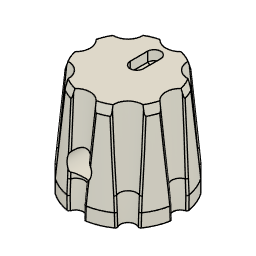
CHORDS Knob 1 (Autodesk Fusion 360 design; units mm, degrees)
Autodesk Fusion 360 part; units mm, degrees
sketch "Sketch1" plane through (0, 0, 0) normal (0, 1, 0) x (1, 0, 0)
  circle A0 centre (0, 0) radius 3
  line L0 (0, 0) -> (0, 3) construction
  line L1 (0, 3) -> (0, -1.6) construction
  line L2 (0, -1.6) -> (-2.5377, -1.6)
  line L3 (0, -1.6) -> (2.5377, -1.6)
  circle A1 centre (0, 0) radius 3.17
  line L4 (0, -1.72) -> (2.5377, -1.72)
  line L5 (0, -1.72) -> (-2.5377, -1.72)
  circle A2 centre (0, 0) radius 4.5
  circle A3 centre (0, 0) radius 6
  line L6 (0, 6) -> (0, 4.5) construction
  circle A4 centre (0, 6) radius 0.875
  circle A5 centre (-4.2426, 4.2426) radius 0.875
  circle A6 centre (-6, 0) radius 0.875
  circle A7 centre (-4.2426, -4.2426) radius 0.875
  circle A8 centre (0, -6) radius 0.875
  circle A9 centre (4.2426, -4.2426) radius 0.875
  circle A10 centre (6, 0) radius 0.875
  line L7 (2.5377, -1.72) -> (2.9, -1.72)
  line L8 (-2.5377, -1.72) -> (-2.8, -1.72)
  circle A11 centre (4.2426, 4.2426) radius 0.875
  line L9 (0, 0) -> (0, 3) construction
  line L10 (-0.75, 3) -> (-0.75, 1)
  arc A12 (-0.75, 1) -> (0.75, 1) centre (0, 1) ccw
  line L11 (0.75, 1) -> (0.75, 3)
  arc A13 (0.75, 3) -> (-0.75, 3) centre (0, 3) ccw
  line L12 (0, 3) -> (0, 1) construction
  dimension "d1" = 6
  dimension "d3" = 4.6
  dimension "d4" = 0.17
  dimension "d5" = 0.12
  dimension "d6" = 9
  dimension "d7" = 1.5
  dimension "d10" = 1.75
  dimension "d12" = 360
  dimension "d62" = 3
  dimension "d63" = 2
  dimension "d64" = 1.5
  constraint coincident A0.centre L0.start
  constraint coincident A0 L0.end
  constraint vertical L0
  constraint parallel L0 L1
  constraint coincident A0 L2.end
  constraint perpendicular L1 L2
  constraint coincident A0 L3.end
  constraint perpendicular L1 L3
  constraint concentric A0 A2
  constraint coincident A3 L6.start
  constraint coincident A2 L6.end
  constraint vertical L6
  constraint coincident L6.start A4.centre
  constraint parallel L4 L7
  constraint parallel L5 L8
  constraint parallel L1 L9
  constraint tangent L10 A12
  constraint tangent A12 L11
  constraint parallel L10 L11
  constraint tangent L11 A13
  constraint tangent L10 A13
  constraint coincident L9 A12.centre
  constraint coincident L0.end L1.start
  measures "d1" diameter of A0
  measures "d3" distance of L0.end L1.end
  measures "d6" diameter of A2
  measures "d10" diameter of A4
  measures "d62" distance of A0.centre L0.end
  measures "d63" distance of L0.end A12.centre
  measures "d64" diameter of A12
extrude "Extrude1" add sketch "Sketch1" along normal blind 10 draft -4.5 contours A0 L2 L3 L10 A12 L11 | A0 A1 L4 L7 L11 A13 | A0 L2 L3 L4 L5 | A0 A1 L4 L5 L7 L8 | A0 L4 L5 | A0 L10 A12 L11 | A0 A1 L10 L11 A13 | A0 A1 L5 L8 L10 A13 | A1 A13 | A2 | A3 A4 A5 A6 A7 A8 A9 A10 A11
sketch "Sketch2" plane through (0, 0, 0) normal (0, 0, 1) x (1, 0, 0)
  line L0 (0, 0) -> (0, 3.2) construction
  circle A0 centre (0, 3.2) radius 1.4
  dimension "d21" = 2.8
  constraint coincident L0.start origin
  constraint vertical L0
  constraint coincident L0.end A0.centre
  measures "d21" diameter of A0
extrude "Extrude5" cut sketch "Sketch1" along normal blind 8 contours A0 L2 L3 L10 A12 L11 | A0 A1 L4 L7 L11 A13 | A0 L2 L3 L4 L5 | A0 L10 A12 L11 | A0 A1 L10 L11 A13 | A0 A1 L5 L8 L10 A13
chamfer "Chamfer2" distance 1 distance2 0.2 8 edges at (4.8162, 10, 1.9949) (1.9949, 10, 4.8162) (-1.9949, 10, 4.8162) (-4.8162, 10, 1.9949) (-4.8162, 10, -1.9949) (-1.9949, 10, -4.8162) (1.9949, 10, -4.8162) (4.8162, 10, -1.9949) measured on face at (5.0774, 6.4078, 2.1031) measured on face at (2.1031, 6.4078, 5.0774) measured on face at (-2.1031, 6.4078, 5.0774) measured on face at (-5.0774, 6.4078, 2.1031) measured on face at (-5.0774, 6.4078, -2.1031) measured on face at (-2.1031, 6.4078, -5.0774) measured on face at (2.1031, 6.4078, -5.0774) measured on face at (5.0774, 6.4078, -2.1031)
extrude "Extrude7" cut sketch "Sketch1" against normal blind 1.5 from surface at 10 contours A0 L10 A12 L11 | A0 A1 L10 L11 A13 | A1 A13
chamfer "Chamfer4" distance 0.4 distance2 0.75 4 edges at (-0.75, 8.5, -2) (0, 8.5, -3.75) (0.75, 8.5, -2) (0, 8.5, -0.25) measured on face at (-0.75, 9.5, -2.3333) measured on face at (0.64, 9, -3.3911) measured on face at (0.75, 9.5, -1.6667) measured on face at (0.5745, 9.5, -0.5179)
extrude "Extrude8" cut sketch "Sketch2" along normal blind 10
extrude "Extrude9" cut sketch "Sketch1" along normal blind 1 contours A0 A1 L4 L5 L7 L8 | A0 L4 L5
chamfer "Chamfer5" distance 0.4 distance2 1 1 edges at (-2.9555, 0, 1.1463) measured on face at (-4.5973, 0, 1.3986)
fillet "Fillet7" radius 1 2 edges at (2.6628, 4.5, 1.72) (-2.6628, 4.5, 1.72)
extrude "Extrude10" add 1 faces at (1.1929, 0, -4.8108) along direction (0, -1, 0) blind 1.5
fillet "Fillet8" radius 40 8 edges at (0, 0, 5.125) (-3.6239, 0, 3.6239) (-5.125, 0, 0) (-3.6239, 0, -3.6239) (0, 0, -5.125) (3.6239, 0, -3.6239) (5.125, 0, 0) (3.6239, 0, 3.6239)
fillet "Fillet3" radius 0.2 50 edges at (3.0348, 5.2493, 4.6908) (3.4859, 0.7834, 4.8076) (1.2253, 6.5121, 5.3489) (0.9973, 1.9012, 5.7647) (0.9346, 0.7833, 5.8643) (-1.2255, 6.515, 5.3487) (-0.9973, 1.9013, 5.7647) (-0.9346, 0.7834, 5.8643) (-3.0357, 5.2413, 4.691) (-3.4859, 0.7833, 4.8076) (-4.6908, 5.2493, 3.0348) (-4.8076, 0.7834, 3.4859) (-5.4635, 5.2413, 1.1705) (-5.8643, 0.7833, 0.9346) (-5.4628, 5.2493, -1.1709) (-5.8643, 0.7834, -0.9346) (-4.691, 5.2413, -3.0357) (-4.8076, 0.7833, -3.4859) (-3.0348, 5.2493, -4.6908) (-3.4859, 0.7834, -4.8076) (-1.1705, 5.2413, -5.4635) (-0.9346, 0.7833, -5.8643) (1.1709, 5.2493, -5.4628) (0.9346, 0.7834, -5.8643) (3.0357, 5.2413, -4.691) (3.4859, 0.7833, -4.8076) (4.6908, 5.2493, -3.0348) (4.8076, 0.7834, -3.4859) (5.4635, 5.2413, -1.1705) (5.8643, 0.7833, -0.9346) (5.4628, 5.2493, 1.1709) (5.8643, 0.7834, 0.9346) (4.691, 5.2413, 3.0357) (4.8076, 0.7833, 3.4859) (3.5737, -0.7499, 4.8196) (0.881, -0.7499, 5.935) (-0.881, -0.7499, 5.935) (-3.5737, -0.7499, 4.8196) (-4.8196, -0.7499, 3.5737) (-5.935, -0.7499, 0.881) (-5.935, -0.7499, -0.881) (-4.8196, -0.7499, -3.5737) (-3.5737, -0.7499, -4.8196) (0.881, -0.7499, -5.935) (-0.881, -0.7499, -5.935) (3.5737, -0.7499, -4.8196) (4.8196, -0.7499, -3.5737) (4.8196, -0.7499, 3.5737) (5.935, -0.7499, 0.881) (5.935, -0.7499, -0.881)
